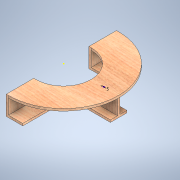
# Autodesk Inventor part: Cuptable1
Saved by Autodesk Inventor 2021 (Build 250183000, 183)
## iProperties
Created: 2021-07-10
Part Number: Cuptable1
Material: Wood (Birch)
Document SubType Name: Modeling
Designer: KAVYA
Density: 0.55 g/cm^3
Appearance: Birch - Natural Polished
Author: KAVYA
Autodesk Inventor part; units mm, degrees
ref_plane "YZ Plane" through (0, 0, 0) normal (1, 0, 0) x (0, 1, 0)
ref_plane "XZ Plane" through (0, 0, 0) normal (0, 1, 0) x (-1, 0, 0)
ref_plane "XY Plane" through (0, 0, 0) normal (0, 0, 1) x (1, 0, 0)
sketch "Sketch1" plane through (0, 0, 0) normal (0, 1, 0) x (-1, 0, 0)
  arc A0 (0, 100) -> (0, -100) centre (0, 0) ccw
  arc A1 (0, 200) -> (0, -200) centre (0, 0) ccw
  line L0 (0, 200) -> (0, 100)
  line L1 (0, -100) -> (0, -200)
  dimension "d0" = 200
  dimension "d1" = 400
  constraints: 4 end point, 4 point on circle, 2 centre point, 2 coincident, 2 vertical
  measures "d0" diameter of A0
  measures "d1" diameter of A1
extrude "Extrusion1" add sketch "Sketch1" along normal blind 8
sketch "Sketch2" plane through (0, 8, 0) normal (0, 1, 0) x (1, 0, 0)
  line L0 (0, -100) -> (0, -200) projected
  line L1 (0, -200) -> (-8, -200)
  line L2 (-8, -200) -> (-8, -100)
  line L3 (-8, -100) -> (0, -100)
  line L4 (0, -100) -> (0, -200)
  line L5 (0, 200) -> (0, 100) projected
  line L6 (0, 100) -> (0, 200)
  line L7 (0, 200) -> (-8, 200)
  line L8 (-8, 200) -> (-8, 100)
  line L9 (-8, 100) -> (0, 100)
  point P0 (0, 0)
  dimension "d4" = 8
  dimension "d5" = 100
  dimension "d6" = 8
  dimension "d7" = 100
  constraints: 16 end point, 3 perpendicular, 1 collinear, 1 horizontal
  measures "d4" distance of L0.end L1.end
  measures "d5" distance of L1.end L2.end
  measures "d6" distance of L5.start L7.end
  measures "d7" distance of L7.end L8.end
extrude "Extrusion2" add sketch "Sketch2" against normal blind 62
sketch "Sketch3" plane through (0, -54, 0) normal (0, -1, 0) x (1, 0, 0)
  line L0 (-8, -100) -> (-8, -200) projected
  line L1 (-8, -200) -> (52, -200)
  line L2 (52, -200) -> (52, -100)
  line L3 (52, -100) -> (-8, -100)
  line L4 (-8, -100) -> (-8, -200)
  line L5 (-8, 200) -> (-8, 100) projected
  line L6 (-8, 100) -> (52, 100)
  line L7 (52, 100) -> (52, 200)
  line L8 (52, 200) -> (-8, 200)
  line L9 (-8, 200) -> (-8, 100)
  point P0 (0, 0)
  dimension "d10" = 60
  dimension "d11" = 60
  constraints: 16 end point, 4 parallel, 2 horizontal, 2 perpendicular
  measures "d10" distance of L3.end L2.end
  measures "d11" distance of L8.end L7.end
extrude "Extrusion3" add sketch "Sketch3" along normal blind 8
sketch "Sketch4" plane through (0, 0, 0) normal (0, -1, 0) x (1, 0, 0)
  arc A0 (0, -100) -> (0, 100) centre (0, 0) ccw projected
  line L0 (100, 0) -> (200, 0)
  line L1 (200, 0) -> (200, 4)
  line L2 (200, 4) -> (100, 4)
  line L3 (100, 4) -> (100, 0)
  line L4 (100, 0) -> (200, 0)
  line L5 (200, 0) -> (200, -4)
  line L6 (200, -4) -> (100, -4)
  line L7 (100, -4) -> (100, 0)
  dimension "d14" = 100
  dimension "d15" = 4
  dimension "d16" = 100
  dimension "d17" = 4
  constraints: 16 end point, 4 parallel, 2 horizontal, 2 perpendicular, 1 point on circle
  measures "d14" distance of L2.end L1.end
  measures "d15" distance of L1.end L0.end
  measures "d16" distance of L5.end L6.end
  measures "d17" distance of L4.end L5.end
extrude "Extrusion4" add sketch "Sketch4" along normal blind 54
sketch "Sketch5" plane through (0, -54, 0) normal (0, -1, 0) x (1, 0, 0)
  line L0 (200, -4) -> (200, 4) projected
  line L1 (200, 0) -> (100, 0)
  line L2 (100, 0) -> (100, -30)
  line L3 (100, -30) -> (200, -30)
  line L4 (200, -30) -> (200, 0)
  line L5 (200, 0) -> (100, 0)
  line L6 (100, 0) -> (100, 30)
  line L7 (100, 30) -> (200, 30)
  line L8 (200, 30) -> (200, 0)
  point P0 (0, 0)
  dimension "d20" = 100
  dimension "d21" = 30
  dimension "d22" = 100
  dimension "d23" = 30
  constraints: 16 end point, 4 parallel, 2 horizontal, 2 perpendicular, 1 midpoint
  measures "d20" distance of L3.end L2.end
  measures "d21" distance of L2.end L1.end
  measures "d22" distance of L6.end L7.end
  measures "d23" distance of L5.end L6.end
extrude "Extrusion5" add sketch "Sketch5" along normal blind 8
sketch "Sketch6" plane through (0, 8, 0) normal (0, 1, 0) x (1, 0, 0)
  circle A0 centre (146.0864, 0) radius 2.5
  point P0 (0, 0)
  dimension "d26" = 5
  constraints: 1 centre point
  measures "d26" diameter of A0
body "Solid1"
